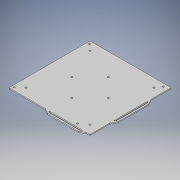
# Autodesk Inventor part: SecondLayer
Saved by Autodesk Inventor 2018 (Build 220112000, 112)
## iProperties
Created: 2019-09-30
Part Number: SecondLayer
Material: Generic
Document SubType Name: Modeling
Designer: anirudh
Density: 1 g/cm^3
Appearance: Default
Author: anirudh
Autodesk Inventor part; units mm, degrees
ref_plane "YZ Plane" through (0, 0, 0) normal (1, 0, 0) x (0, 1, 0)
ref_plane "XZ Plane" through (0, 0, 0) normal (0, 1, 0) x (-1, 0, 0)
ref_plane "XY Plane" through (0, 0, 0) normal (0, 0, 1) x (1, 0, 0)
sketch "Sketch1" plane through (0, 0, 0) normal (0, 1, 0) x (-1, 0, 0)
  circle A0 centre (158.4676, -17.4724) radius 1.75
  circle A1 centre (158.4676, -174.9524) radius 1.75
  circle A2 centre (3.5476, -174.9524) radius 1.75
  circle A3 centre (26.3876, -17.4724) radius 1.75
  line L0 (-6.6324, -13.1224) -> (-6.6324, -179.3024)
  line L1 (-4.6324, -181.3024) -> (161.5476, -181.3024)
  line L2 (163.5476, -179.3024) -> (163.5476, -13.1224)
  line L3 (161.5476, -11.1224) -> (-4.6324, -11.1224)
  arc A4 (-4.6324, -11.1224) -> (-6.6324, -13.1224) centre (-4.6324, -13.1224) ccw
  arc A5 (-4.6324, -11.1224) -> (-6.6324, -13.1224) centre (-4.6324, -13.1224) ccw
  arc A6 (163.5476, -13.1224) -> (161.5476, -11.1224) centre (161.5476, -13.1224) ccw
  arc A7 (163.5476, -13.1224) -> (161.5476, -11.1224) centre (161.5476, -13.1224) ccw
  arc A8 (161.5476, -181.3024) -> (163.5476, -179.3024) centre (161.5476, -179.3024) ccw
  arc A9 (161.5476, -181.3024) -> (163.5476, -179.3024) centre (161.5476, -179.3024) ccw
  arc A10 (-6.6324, -179.3024) -> (-4.6324, -181.3024) centre (-4.6324, -179.3024) ccw
  arc A11 (-6.6324, -179.3024) -> (-4.6324, -181.3024) centre (-4.6324, -179.3024) ccw
  circle A12 centre (78.4576, -58.1124) radius 1.75
  circle A13 centre (116.5576, -96.2124) radius 1.75
  circle A14 centre (78.4576, -134.3124) radius 1.75
  circle A15 centre (40.3576, -96.2124) radius 1.75
  line L4 (154.6576, -20.0124) -> (167.3576, -20.0124) construction
  line L5 (2.2576, -20.0124) -> (14.9576, -20.0124) construction
  circle A16 centre (145.6773, -28.9927) radius 1.75
  circle A17 centre (11.2378, -28.9927) radius 1.75
  circle A18 centre (11.2378, -163.4322) radius 1.75
  circle A19 centre (145.6773, -163.4322) radius 1.75
  point P0 (0, 0)
  dimension "d1" = 3.5
  dimension "d2" = 3.5
  dimension "d3" = 3.5
  dimension "d18" = 3.5
  dimension "d19" = 3.5
  dimension "d21" = 3.5
  dimension "d28" = 3.5
  dimension "d30" = 3.5
  dimension "d31" = 3.5
  constraints: 22 point on circle, 20 centre point, 12 end point, 5 coincident, 4 point on line, 2 horizontal, 2 parallel, 1 perpendicular
  measures "d1" diameter of A1
  measures "d2" diameter of A2
  measures "d3" diameter of A3
  measures "d18" diameter of A12
  measures "d19" diameter of A13
  measures "d21" diameter of A15
  measures "d28" diameter of A16
  measures "d30" diameter of A18
  measures "d31" diameter of A19
extrude "Extrusion2" add sketch "Sketch1" along normal blind 2.286
sketch "Sketch3" plane through (0, 2.286, 0) normal (0, 1, 0) x (1, 0, 0)
  line L0 (12.9824, 96.2124) -> (12.9824, 127.9624)
  line L1 (12.9824, 96.2124) -> (12.9824, 64.4624)
  line L2 (12.9824, 64.4624) -> (6.6324, 52.6096)
  line L3 (6.6324, 139.8153) -> (12.9824, 127.9624)
  arc A0 (9.8074, 127.9624) -> (6.6324, 131.1374) centre (6.6324, 127.9624) ccw
  arc A1 (6.6324, 61.2874) -> (9.8074, 64.4624) centre (6.6324, 64.4624) ccw
  line L4 (9.8074, 127.9624) -> (9.8074, 64.4624)
  line L5 (6.6324, 52.6096) -> (6.6324, 61.2874)
  line L6 (6.6324, 131.1374) -> (6.6324, 139.8153)
  line L7 (6.6324, 139.8153) -> (6.6324, 131.1374)
  line L8 (6.6324, 61.2874) -> (6.6324, 52.6096)
  line L9 (-43.6028, 4.7724) -> (-11.8528, 4.7724)
  line L10 (-43.6028, 4.7724) -> (-75.3528, 4.7724)
  line L11 (-75.3528, 4.7724) -> (-87.2056, 11.1224)
  line L12 (0, 11.1224) -> (-11.8528, 4.7724)
  arc A2 (-11.8528, 7.9474) -> (-8.6778, 11.1224) centre (-11.8528, 11.1224) ccw
  arc A3 (-78.5278, 11.1224) -> (-75.3528, 7.9474) centre (-75.3528, 11.1224) ccw
  line L13 (-11.8528, 7.9474) -> (-75.3528, 7.9474)
  line L14 (-8.6778, 11.1224) -> (0, 11.1224)
  line L15 (-78.5278, 11.1224) -> (-87.2056, 11.1224)
  point P0 (0, 0)
  point P1 (6.6324, 13.1224)
  point P2 (6.6324, 179.3024)
  point P3 (-161.5476, 11.1224)
  constraints: 32 end point, 8 point on circle, 4 centre point, 3 parallel
extrude "Extrusion5" add sketch "Sketch3" against normal blind 2.286
body "Solid2"
